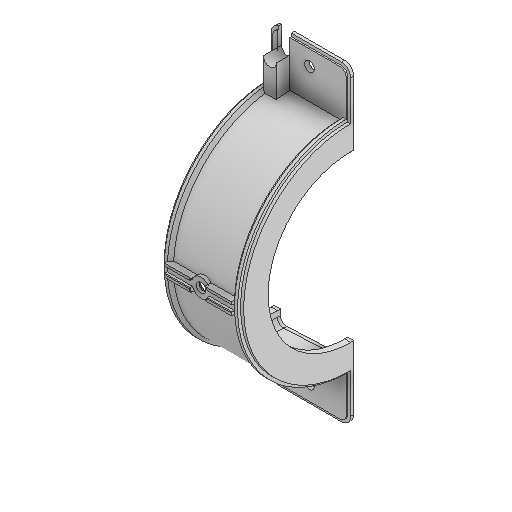
# Autodesk Inventor part: Test
Saved by Autodesk Inventor 2025.2 (Build 292293000, 293)
## iProperties
Created: 2025-04-17
Part Number: Test
Material: Generic
Document SubType Name: Modeling
Designer: Andreas
Density: 1 g/cm^3
Appearance: Default
Author: Andreas
Autodesk Inventor part; units mm, degrees
ref_plane "YZ Plane" through (0, 0, 0) normal (1, 0, 0) x (0, 1, 0)
ref_plane "XZ Plane" through (0, 0, 0) normal (0, 1, 0) x (-1, 0, 0)
ref_plane "XY Plane" through (0, 0, 0) normal (0, 0, 1) x (1, 0, 0)
sketch "Sketch1" plane through (0, 0, 0) normal (0, 0, 1) x (1, 0, 0)
  line L0 (0, 30) -> (0, 31.907)
  line L1 (2.0908, 33.905) -> (18, 33.1818)
  line L2 (22, 29.5) -> (22, 27)
  line L3 (22, 27) -> (24, 27)
  line L4 (24, 27) -> (24, 35)
  line L5 (-2, 35) -> (-2, 30)
  line L6 (-2, 30) -> (0, 30)
  line L7 (0, 0) -> (88.4682, 0)
  arc A0 (2.0908, 33.905) -> (0, 31.907) centre (2, 31.907) ccw
  line L8 (18, 33.1818) -> (22, 29.5)
  line L9 (-2, 35) -> (-1, 35)
  line L10 (-1, 35) -> (-1, 36)
  line L11 (-1, 36) -> (0, 36)
  line L12 (0, 36) -> (0, 35)
  line L13 (0, 35) -> (22, 35)
  line L14 (22, 35) -> (22, 36)
  line L15 (24, 35) -> (23, 35)
  line L16 (23, 35) -> (23, 36)
  line L17 (23, 36) -> (22, 36)
  point P0 (0, 34)
  point P1 (22, 33)
  point P2 (-1, 30)
  point P3 (22.5, 36)
  point P4 (-0.5, 36)
  dimension "d0" = 66
  dimension "d1" = 68
  dimension "d2" = 22
  dimension "d3" = 2
  dimension "d4" = 6
  dimension "d7" = 2
  dimension "d8" = 4
  dimension "d9" = 3.5
  dimension "d10" = 4
  dimension "d11" = 2
  dimension "d12" = 1
  dimension "d13" = 70
  dimension "d14" = 1
  dimension "d16" = 26
  constraints: 36 end point, 8 perpendicular, 5 equal length, 4 horizontal, 4 point on line, 3 midpoint, 3 vertical, 2 point on circle, 2 tangent, 1 centre point, 1 horizontal alignment, 1 parallel, 1 vertical alignment
  measures "d0" diameter of point (22, 33) L7
  measures "d1" diameter of point (0, 34) L7
  measures "d2" horizontal distance of point (0, 34) point (22, 33)
  measures "d3" distance of L2.end L3.end
  measures "d4" distance from line of point (22, 33) L3
  measures "d7" radius of A0
  measures "d8" horizontal distance of L1.end point (22, 33)
  measures "d9" distance of L2.start point (22, 33)
  measures "d10" vertical distance of point (0, 34) point (-1, 30)
  measures "d11" distance of L5.end L0.start
  measures "d12" distance of L5.start L9.end
  measures "d13" diameter of L9 L7
  measures "d14" distance of L11.end L12.end
  measures "d16" distance between parallel lines of L4 L5
revolve "Revolution1" add sketch "Sketch1" angle 180 about axis through (0, 0, 0) along (1, 0, 0)
sketch "Sketch2" plane through (22, -35, 0) normal (0, 0, -1) x (-1, 0, 0)
  line L0 (24, 0) -> (24, 5) projected
  line L1 (24, 0) -> (-2, 0)
  line L2 (-2, 0) -> (-2, -13)
  line L3 (1, -16) -> (21, -16)
  line L4 (24, -13) -> (24, 0)
  arc A0 (21, -16) -> (24, -13) centre (21, -13) ccw
  arc A1 (-2, -13) -> (1, -16) centre (1, -13) ccw
  line L5 (24, 5) -> (22, 5) projected
  line L6 (22, 5) -> (22, 3.093) projected
  arc A2 (19.9092, 1.095) -> (22, 3.093) centre (20, 3.093) ccw projected
  line L7 (19.9092, 1.095) -> (4, 1.8182) projected
  line L8 (4, 1.8182) -> (0, 5.5) projected
  line L9 (0, 5.5) -> (0, 8) projected
  line L10 (0, 8) -> (-2, 8) projected
  line L11 (-2, 8) -> (-2, 0) projected
  line L12 (-2, 0) -> (-1, 0) projected
  line L13 (-1, 0) -> (-1, -1) projected
  line L14 (-1, -1) -> (0, -1) projected
  line L15 (0, -1) -> (0, 0) projected
  line L16 (0, 0) -> (22, 0) projected
  line L17 (22, 0) -> (22, -1) projected
  line L18 (22, -1) -> (23, -1) projected
  line L19 (23, -1) -> (23, 0) projected
  line L20 (23, 0) -> (24, 0) projected
  line L21 (24, 0) -> (24, 5) projected
  point P0 (22, 35)
  dimension "d17" = 51
  dimension "d18" = 3
  constraints: 8 end point, 4 point on circle, 4 tangent, 2 centre point, 2 parallel, 1 coincident, 1 equal radius, 1 horizontal, 1 perpendicular
  measures "d17" distance from line of point (22, 35) L3
  measures "d18" radius of A0
extrude "Extrusion1" add sketch "Sketch2" along normal blind 1
sketch "Sketch3" plane through (22, -35, 0) normal (0, 0, 1) x (1, 0, 0)
  line L0 (-24, -13) -> (-24, 0) projected
  arc A0 (-24, -13) -> (-21, -16) centre (-21, -13) ccw projected
  line L1 (-1, -16) -> (-21, -16) projected
  arc A1 (-1, -16) -> (2, -13) centre (-1, -13) ccw projected
  line L2 (2, 0) -> (2, -13) projected
  line L3 (0, 0) -> (-22, 0) projected
  line L4 (0, -1) -> (0, 71) projected
  line L5 (-22, -1) -> (-22, 71) projected
  line L6 (-23, 0) -> (-23, -13)
  arc A2 (-23, -13) -> (-21, -15) centre (-21, -13) ccw
  line L7 (-21, -15) -> (-1, -15)
  arc A3 (-1, -15) -> (1, -13) centre (-1, -13) ccw
  line L8 (1, -13) -> (1, 0)
  line L9 (-22, -1) -> (-23, -1) projected
  line L10 (1, -1) -> (0, -1) projected
  point P0 (-22, 35)
  constraints: 6 end point, 4 point on circle, 2 centre point, 1 point on line, 4 other
extrude "Extrusion2" add sketch "Sketch3" along normal blind 0.5
sketch "Sketch4" plane through (22, -35, -1) normal (0, 0, -1) x (-1, 0, 0)
  line L0 (1, -16) -> (21, -16) projected
  point P0 (22, 35)
  point P1 (11, -10)
  point P2 (11, -16)
  dimension "d30" = 45
  constraints: 1 midpoint, 1 vertical alignment
  measures "d30" vertical distance of point (22, 35) point (11, -10)
hole "Hole1" at (11, -45, -1) direction (0, 0, 1) diameter 3.2 depth 4.5 tip angle 118
mirror "Mirror1" about plane through (0, 0, 0) normal (0, 1, 0) of "Extrusion1", "Extrusion2", "Hole1"
sketch "Sketch5" plane through (21, 51, -1) normal (0, 0, -1) x (-1, 0, 0)
  line L0 (23, -3) -> (23, -21) projected
  line L1 (0, 0) -> (20, 0) projected
  point P0 (21, -51)
  point P1 (18.5, -6)
  dimension "d38" = 4.5
  dimension "d39" = 6
  measures "d38" distance from line of L0 point (18.5, -6)
  measures "d39" distance from line of L1 point (18.5, -6)
hole "Hole2" at (2.5, 45, -1) direction (0, 0, 1) diameter 4.2 depth 8 tip angle 118
chamfer "Chamfer1" distance 1 angle 45 2 edges at (22, 0, 35) (0, 0, 35)
sketch "Sketch6" plane through (0, 35, 0.5) normal (0, 0, 1) x (1, 0, 0)
  circle A0 centre (2.5, 10) radius 2.1 projected
  line L0 (4.6, 10) -> (0.4, 10)
  line L1 (0.4, 10) -> (0.4, -1.0182)
  line L2 (0.4, -1.0182) -> (4.6, -1.2091)
  line L3 (4.6, -1.2091) -> (4.6, 10)
  line L4 (22, 0) -> (0, 0) projected
  line L5 (2.0908, -1.095) -> (18, -1.8182) projected
  point P0 (0, -35)
  point P1 (0.4, 10)
  constraints: 8 end point, 2 point on line, 2 vertical, 1 horizontal, 1 parallel, 1 perpendicular, 2 other
extrude "Extrusion3" add sketch "Sketch6" along normal blind 4.5 contours L3 L4 L1 A0 | L3 L2 L1 L4
sketch "Sketch7" plane through (1, 50, 0.5) normal (0, 0, 1) x (1, 0, 0)
  line L0 (3.6, -15.359) -> (3.6, -5) projected
  line L1 (3.6, -5) -> (-0.6, -5)
  line L2 (-0.6, -5) -> (-0.6, 4.3267)
  line L3 (-0.6, 4.3267) -> (3.6, 4.3267)
  line L4 (3.6, 4.3267) -> (3.6, -5)
  point P0 (-1, -50)
  constraints: 8 end point, 2 parallel, 1 horizontal, 1 perpendicular
extrude "Extrusion4" cut sketch "Sketch7" against normal blind 4.5
ref_plane "Work Plane1" through (-1, 0, 36) normal (0, 0, 1) x (1, 0, 0)
sketch "Sketch8" plane through (-1, 0, 36) normal (0, 0, 1) x (1, 0, 0)
  line L0 (1, -30) -> (1, 30) projected
  line L1 (23, -35.9965) -> (23, 35.9965) projected
  line L2 (1, 2) -> (23, 2)
  line L3 (23, 2) -> (23, -2)
  line L4 (23, -2) -> (1, -2)
  line L5 (1, -2) -> (1, 2)
  circle A0 centre (12, 0) radius 3
  line L6 (1, -35.9965) -> (1, 35.9965) projected
  point P0 (1, 0)
  point P1 (1, 0)
  point P2 (12, -2)
  point P3 (1, 0)
  point P4 (14.2361, -2)
  point P5 (14.2361, 2)
  point P6 (9.7639, 2)
  point P7 (9.7639, -2)
  dimension "d47" = 4
  dimension "d48" = 6
  constraints: 8 end point, 3 midpoint, 2 parallel, 2 point on line, 1 centre point, 1 horizontal, 1 horizontal alignment, 1 perpendicular, 1 vertical alignment, 2 other
  measures "d47" distance between parallel lines of L2 L4
  measures "d48" diameter of A0
extrude "Extrusion5" add sketch "Sketch8" against normal blind 2
sketch "Sketch9" plane through (-1, 0, 36) normal (0, 0, 1) x (1, 0, 0)
  line L0 (23, -2) -> (23, 0) projected
  line L1 (23, 0) -> (23, 2) projected
  line L2 (23, 2) -> (14.2361, 2) projected
  arc A0 (14.2361, 2) -> (9.7639, 2) centre (12, 0) ccw projected
  line L3 (9.7639, 2) -> (1, 2) projected
  line L4 (1, 2) -> (1, 0) projected
  line L5 (1, 0) -> (1, -2) projected
  line L6 (1, -2) -> (9.7639, -2) projected
  arc A1 (9.7639, -2) -> (14.2361, -2) centre (12, 0) ccw projected
  line L7 (14.2361, -2) -> (23, -2) projected
  line L8 (1, 1) -> (23, 1)
  line L9 (23, 1) -> (23, -1)
  line L10 (23, -1) -> (1, -1)
  line L11 (1, -1) -> (1, 1)
  circle A2 centre (12, 0) radius 3
  point P0 (1, 0)
  point P1 (14.8284, 1)
  point P2 (14.8284, -1)
  point P3 (14.2361, -2)
  point P4 (9.1716, 1)
  point P5 (9.7639, 2)
  point P6 (9.1716, -1)
  constraints: 8 end point, 2 midpoint, 2 parallel, 1 coincident, 1 horizontal, 1 perpendicular, 3 other
extrude "Extrusion6" add sketch "Sketch9" along normal blind 1 contours L7 A2 L10 L0 | L6 L5 L10 A2 | L8 A2 L2 L1 | L8 L4 L3 A2
chamfer "Chamfer2" distance 0.2 angle 45 8 edges at (17.9142, 1, 37) (17.9142, -1, 37) (4.0858, -1, 37) (4.0858, 1, 37) (8.4189, 1.529, 37) (8.4189, -1.529, 37) (13.5811, -1.529, 37) (13.5811, 1.529, 37)
sketch "Sketch10" plane through (-1, 0, 36) normal (0, 0, 1) x (1, 0, 0)
  arc A0 (14.2361, 2) -> (9.7639, 2) centre (12, 0) ccw projected
  point P0 (1, 0)
  constraints: 1 coincident
hole "Hole3" at (11, 0, 36) direction (0, 0, -1) diameter 3 end through all
chamfer "Chamfer3" distance 1.5 angle 45 1 edges at (10.9982, 1.5, 33.4665)
body "Solid1"
